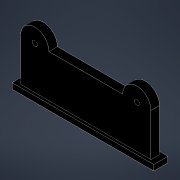
# Autodesk Inventor part: Base
Saved by Autodesk Inventor 2021.2 (Build 252289000, 289)
## iProperties
Created: 2021-05-30
Part Number: Base
Material: Типовые
Document SubType Name: Modeling
Designer: Admin
Density: 1 g/cm^3
Appearance: Черная
Author: Admin
Autodesk Inventor part; units mm, degrees
ref_plane "YZ Plane" through (0, 0, 0) normal (1, 0, 0) x (0, 1, 0)
ref_plane "XZ Plane" through (0, 0, 0) normal (0, 1, 0) x (-1, 0, 0)
ref_plane "XY Plane" through (0, 0, 0) normal (0, 0, 1) x (1, 0, 0)
sketch "Эскиз1" plane through (0, 0, 0) normal (0, 1, 0) x (-1, 0, 0)
  line L0 (0, 0) -> (-500, 0)
  line L1 (-500, 0) -> (-500, -50)
  line L2 (-500, -50) -> (0, -50)
  line L3 (0, -50) -> (0, 0)
  dimension "d0" = 500
  dimension "d1" = 50
  constraints: 8 end point, 2 parallel, 1 horizontal, 1 perpendicular
  measures "d0" distance of L2.end L1.end
  measures "d1" distance of L1.end L0.end
extrude "Выдавливание1" add sketch "Эскиз1" along normal blind 20
sketch "Эскиз3" plane through (0, 20, 0) normal (0, 1, 0) x (1, 0, 0)
  line L0 (20, 40) -> (480, 40)
  line L1 (480, 40) -> (480, 10)
  line L2 (480, 10) -> (20, 10)
  line L3 (20, 10) -> (20, 40)
  line L4 (500, 50) -> (0, 50) projected
  line L5 (0, 0) -> (500, 0) projected
  line L6 (0, 50) -> (0, 0) projected
  line L7 (500, 0) -> (500, 50) projected
  dimension "d8" = 10
  dimension "d9" = 10
  dimension "d10" = 20
  dimension "d11" = 20
  constraints: 8 end point, 2 parallel, 1 horizontal, 1 perpendicular
  measures "d8" distance between parallel lines of L4 L0
  measures "d9" distance between parallel lines of L5 L2
  measures "d10" distance between parallel lines of L6 L3
  measures "d11" distance between parallel lines of L7 L1
extrude "Выдавливание3" add sketch "Эскиз3" along normal blind 150 contours L0 L1 L2 L3
sketch "Эскиз4" plane through (20, 20, -10) normal (0, 0, 1) x (1, 0, 0)
  arc A0 (100, 150) -> (0, 150) centre (50, 150) ccw
  line L0 (0, 150) -> (460, 150) projected
  line L1 (0, 0) -> (0, 150) projected
  line L2 (230, 150) -> (230, 234.7508)
  arc A1 (460, 150) -> (360, 150) centre (410, 150) ccw
  point P0 (-20, -20)
  dimension "d14" = 100
  constraints: 4 point on circle, 3 end point, 2 centre point, 2 point on line, 2 symmetric about line, 1 midpoint, 1 tangent, 1 vertical, 1 other
  measures "d14" diameter of A0
extrude "Выдавливание4" add sketch "Эскиз4" against normal up to surface (30 mm away)
sketch "Эскиз5" plane through (20, 20, -10) normal (0, 0, 1) x (1, 0, 0)
  arc A0 (100, 150) -> (0, 150) centre (50, 150) ccw projected
  arc A1 (460, 150) -> (360, 150) centre (410, 150) ccw projected
  point P0 (-20, -20)
  constraints: 2 coincident
hole "Отверстие1" at (70, 170, -10) at (430, 170, -10) direction (0, 0, -1) diameter 18 end through all
